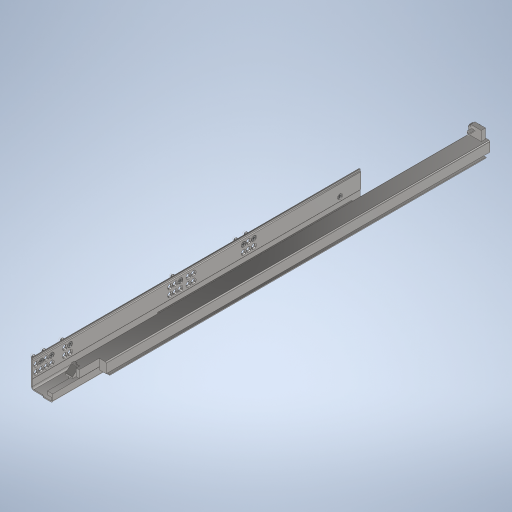
# Autodesk Inventor part: 566H7500B01 Chipboard screws 661.1450.HG 6,3x14,5 top_row L
Saved by Autodesk Inventor 2024 (Build 280153000, 153)
## iProperties
Created: 2019-09-04
Part Number: 566H7500B01 Chipboard screws 661.1450.HG 6,3x14,5 top_row L
Material: Generic
Document SubType Name: Modeling
Designer: RokasM
Density: 1 g/cm^3
Appearance: Default
Author: RokasM
Autodesk Inventor part; units mm, degrees
ref_plane "WP_runner_bottom_displacement_from_facade" through (0, 2, 0) normal (0, 1, 0) x (-1, 0, 0)
sketch "Sketch4" plane through (0, 2, 0) normal (0, 1, 0) x (-1, 0, 0)
  line L0 (0, 47.5) -> (0, 4.8)
  arc A0 (-4.8, 0) -> (0, 4.8) centre (-4.8, 4.8) ccw
  line L1 (-4.8, 0) -> (-36.5, 0)
  arc A1 (-39.3, 2.8) -> (-36.5, 0) centre (-36.5, 2.8) ccw
  line L2 (-39.3, 2.8) -> (-39.3, 13.6)
  line L3 (-39.3, 13.6) -> (-37.5, 13.6)
  line L4 (-37.5, 13.6) -> (-37.5, 2.8)
  arc A2 (-37.5, 2.8) -> (-36.5, 1.8) centre (-36.5, 2.8) ccw
  line L5 (-36.5, 1.8) -> (-4.8, 1.8)
  arc A3 (-4.8, 1.8) -> (-1.8, 4.8) centre (-4.8, 4.8) ccw
  line L6 (-1.8, 4.8) -> (-1.8, 15.95)
  line L7 (-1.8, 15.95) -> (-2.8, 17.25)
  line L8 (-2.8, 17.25) -> (-2.8, 43.75)
  line L9 (-2.8, 43.75) -> (-1.8, 45.05)
  line L10 (-1.8, 45.05) -> (-1.8, 47.5)
  line L11 (-1.8, 47.5) -> (0, 47.5)
  point P0 (0, 0)
  point P1 (-20.65, 0)
  point P2 (0, 26.15)
  dimension "d54" = 2.8
  dimension "d55" = 4.8
  dimension "d56" = 3
  dimension "d57" = 1
  dimension "d58" = 39.3
  dimension "d59" = 47.5
  dimension "d60" = 13.6
  dimension "d61" = 26.5
  dimension "d62" = 2.45
  dimension "d63" = 11.15
  dimension "d64" = 1
  constraints: 24 end point, 8 point on circle, 6 tangent, 5 parallel, 4 centre point, 4 perpendicular, 2 concentric, 2 equal length, 2 midpoint, 1 horizontal, 1 horizontal alignment, 1 vertical alignment
  measures "d54" radius of A1
  measures "d55" radius of A0
  measures "d56" radius of A3
  measures "d57" radius of A2
  measures "d58" distance between parallel lines of L2 L0
  measures "d59" distance between parallel lines of L11 L1
  measures "d60" distance between parallel lines of L3 L1
  measures "d61" distance of L7.end L8.end
  measures "d62" distance of L9.end L10.end
  measures "d63" distance of L6.start L6.end
  measures "d64" distance between parallel lines of L10 L8
extrude "0101_runner_bottom" add sketch "Sketch4" along normal blind 574.8
sketch "Sketch5" plane through (37.5, 2, 2.8) normal (-1, 0, 0) x (0, 0, 1)
  line L0 (10.8, 87) -> (4.9, 87)
  line L1 (4.9, 87) -> (4.9, 0)
  line L2 (4.9, 0) -> (10.8, 0)
  line L3 (10.8, 0) -> (10.8, 87)
  line L4 (10.8, 0) -> (0, 0) projected
  line L5 (10.8, 0) -> (10.8, 574.8) projected
  point P0 (-2.8, -2)
  dimension "d67" = 5.9
  dimension "d68" = 87
  constraints: 8 end point, 2 collinear, 2 parallel, 1 horizontal, 1 perpendicular
  measures "d67" distance of L2.end L1.end
  measures "d68" distance of L1.end L0.end
extrude "0102_runner_bottom_edge" add sketch "Sketch5" along normal blind 7.2
ref_plane "WP_cylinder_start" through (0, 328.35, 0) normal (0, -1, 0) x (1, 0, 0)
sketch "Sketch17" plane through (0, 328.35, 0) normal (0, -1, 0) x (1, 0, 0)
  line L0 (13.3, 1.8) -> (13.3, 6.125)
  arc A0 (21.8, 6.125) -> (13.3, 6.125) centre (17.55, 6.125) ccw
  line L1 (21.8, 6.125) -> (21.8, 3.325)
  line L2 (21.8, 3.325) -> (25, 3.325)
  line L3 (25, 3.325) -> (25, 1.8)
  line L4 (25, 1.8) -> (13.3, 1.8)
  line L5 (4.8, 1.8) -> (36.5, 1.8) projected
  line L6 (0, 4.8) -> (0, 47.5) projected
  point P0 (0, 0)
  dimension "d143" = 4.25
  dimension "d144" = 13.3
  dimension "d145" = 1.525
  dimension "d146" = 3.2
  dimension "d147" = 4.325
  constraints: 10 end point, 4 perpendicular, 2 point on circle, 2 tangent, 1 centre point, 1 collinear
  measures "d143" radius of A0
  measures "d144" distance between parallel lines of L6 L0
  measures "d145" distance between parallel lines of L4 L2
  measures "d146" distance between parallel lines of L1 L3
  measures "d147" distance from line of L4 A0.centre
extrude "0104_cylinder" add sketch "Sketch17" against normal blind 147.5
sketch "Sketch18" plane through (0, 328.35, 0) normal (0, -1, 0) x (1, 0, 0)
  circle A0 centre (17.55, 6.125) radius 0.99
  arc A1 (21.8, 6.125) -> (13.3, 6.125) centre (17.55, 6.125) ccw projected
  point P0 (0, 0)
  point P1 (14.5149, 9.1)
  dimension "d150" = 1.98
  constraints: 1 centre point, 1 concentric
  measures "d150" diameter of A0
extrude "0105_cylinder_piston" add sketch "Sketch18" along normal blind 5.293
sketch "Sketch19" plane through (17.55, 323.057, 6.125) normal (0, -1, 0) x (1, 0, 0)
  line L0 (-3.02, 1.475) -> (4.33, 1.475)
  line L1 (4.33, 1.475) -> (4.33, -4.325)
  line L2 (4.33, -4.325) -> (-3.02, -4.325)
  line L3 (-3.02, -4.325) -> (-3.02, 1.475)
  line L4 (-12.75, -4.325) -> (18.95, -4.325) projected
  line L5 (-17.55, -1.325) -> (-17.55, 41.375) projected
  point P0 (-17.55, -6.125)
  dimension "d153" = 7.35
  dimension "d154" = 5.8
  dimension "d155" = 21.88
  constraints: 8 end point, 2 parallel, 1 collinear, 1 horizontal, 1 perpendicular
  measures "d153" distance between parallel lines of L1 L3
  measures "d154" distance between parallel lines of L2 L0
  measures "d155" distance between parallel lines of L5 L1
extrude "010601_piston_support" add sketch "Sketch19" along normal blind 29.35
sketch "Sketch20" plane through (14.53, 323.057, 7.6) normal (0, 0, 1) x (1, 0, 0)
  line L0 (0.22, -11.475) -> (6.72, -11.475)
  line L1 (6.72, -11.475) -> (6.72, -17.975)
  line L2 (6.72, -17.975) -> (0.22, -17.975)
  line L3 (0.22, -17.975) -> (0.22, -11.475)
  line L4 (7.35, 0) -> (7.35, -29.35) projected
  line L5 (7.35, 0) -> (0, 0) projected
  point P0 (-14.53, -323.057)
  dimension "d158" = 6.5
  dimension "d159" = 6.5
  dimension "d332" = 0.63
  dimension "d333" = 11.475
  constraints: 8 end point, 2 parallel, 1 horizontal, 1 perpendicular
  measures "d158" distance between parallel lines of L2 L0
  measures "d159" distance between parallel lines of L1 L3
  measures "d332" distance between parallel lines of L4 L1
  measures "d333" distance between parallel lines of L5 L0
extrude "010602_piston_support_extrusion" add sketch "Sketch20" along normal blind 4.125
ref_plane "WP_runner_top_displacement_from_runner_bottom" through (0, 48.5, 0) normal (0, -1, 0) x (1, 0, 0)
sketch "Sketch6" plane through (0, 48.5, 0) normal (0, -1, 0) x (1, 0, 0)
  line L0 (33.65, 26.525) -> (38.95, 26.525)
  line L1 (38.95, 26.525) -> (38.95, 13.6)
  line L2 (38.95, 13.6) -> (33.65, 13.6)
  line L3 (33.65, 13.6) -> (33.65, 26.525)
  line L4 (39.3, 13.6) -> (39.3, 2.8) projected
  line L5 (30.3, 13.6) -> (39.3, 13.6) projected
  point P0 (0, 0)
  dimension "d72" = 5.3
  dimension "d73" = 12.925
  dimension "d74" = 0.35
  constraints: 8 end point, 2 parallel, 1 collinear, 1 horizontal, 1 perpendicular
  measures "d72" distance of L1.end L2.end
  measures "d73" distance of L0.end L1.end
  measures "d74" distance between parallel lines of L4 L1
extrude "0201_runner_top" add sketch "Sketch6" against normal blind 35 separate body
sketch "Sketch7" plane through (0, 83.5, 0) normal (0, 1, 0) x (1, 0, 0)
  line L0 (51.05, -26.525) -> (21.35, -26.525)
  line L1 (21.35, -26.525) -> (21.35, -9.125)
  line L2 (21.35, -9.125) -> (51.05, -9.125)
  line L3 (51.05, -9.125) -> (51.05, -26.525)
  line L4 (38.95, -26.525) -> (38.95, -13.6) projected
  line L5 (33.65, -26.525) -> (38.95, -26.525) projected
  point P0 (0, 0)
  dimension "d77" = 29.7
  dimension "d78" = 17.4
  dimension "d79" = 12.1
  constraints: 8 end point, 2 parallel, 1 collinear, 1 horizontal, 1 perpendicular
  measures "d77" distance of L1.end L2.end
  measures "d78" distance of L0.end L1.end
  measures "d79" distance between parallel lines of L4 L3
extrude "0202_runner_top" add sketch "Sketch7" along normal blind 668 bodies 2
sketch "Sketch8" plane through (0, 83.5, 0) normal (0, -1, 0) x (1, 0, 0)
  line L0 (21.35, 9.125) -> (21.35, 26.525)
  line L1 (21.35, 26.525) -> (33.65, 26.525)
  line L2 (33.65, 26.525) -> (33.65, 13.6)
  line L3 (33.65, 13.6) -> (30.3, 13.6)
  line L4 (30.3, 13.6) -> (30.3, 9.125)
  line L5 (30.3, 9.125) -> (21.35, 9.125)
  line L6 (21.35, 26.525) -> (33.65, 26.525) projected
  line L7 (33.65, 26.525) -> (33.65, 13.6) projected
  line L8 (30.3, 13.6) -> (39.3, 13.6) projected
  line L9 (30.3, 7.7) -> (30.3, 13.6) projected
  line L10 (51.05, 9.125) -> (21.35, 9.125) projected
  line L11 (21.35, 9.125) -> (21.35, 26.525) projected
  point P0 (0, 0)
  constraints: 12 end point, 6 collinear
extrude "0203_runner_top" add sketch "Sketch8" along normal blind 26.1 bodies 2
sketch "Sketch9" plane through (0, 57.4, 0) normal (0, -1, 0) x (1, 0, 0)
  line L0 (26.75, 26.525) -> (33.65, 26.525)
  line L1 (33.65, 26.525) -> (33.65, 13.6)
  line L2 (33.65, 13.6) -> (30.3, 13.6)
  line L3 (30.3, 13.6) -> (30.3, 9.125)
  line L4 (30.3, 9.125) -> (26.75, 9.125)
  line L5 (26.75, 9.125) -> (26.75, 26.525)
  line L6 (33.65, 26.525) -> (21.35, 26.525) projected
  line L7 (33.65, 26.525) -> (33.65, 13.6) projected
  line L8 (30.3, 13.6) -> (39.3, 13.6) projected
  line L9 (30.3, 7.7) -> (30.3, 13.6) projected
  line L10 (21.35, 9.125) -> (30.3, 9.125) projected
  point P0 (0, 0)
  dimension "d84" = 6.9
  constraints: 12 end point, 5 collinear, 1 parallel
  measures "d84" distance between parallel lines of L1 L5
extrude "0204_runner_top" add sketch "Sketch9" along normal blind 2.5 bodies 2
sketch "Sketch10" plane through (33.65, 48.5, 26.525) normal (0, 0, 1) x (1, 0, 0)
  line L0 (-10.8, 701.485) -> (11.2, 701.485)
  line L1 (11.2, 701.485) -> (11.2, 694)
  line L2 (11.2, 694) -> (-10.8, 694)
  line L3 (-10.8, 694) -> (-10.8, 701.485)
  line L4 (-12.3, 703) -> (17.4, 703) projected
  line L5 (17.4, 35) -> (17.4, 703) projected
  point P0 (-33.65, -48.5)
  dimension "d87" = 22
  dimension "d88" = 7.485
  dimension "d89" = 1.515
  dimension "d90" = 6.2
  constraints: 8 end point, 2 parallel, 1 horizontal, 1 perpendicular
  measures "d87" distance of L1.end L2.end
  measures "d88" distance of L0.end L1.end
  measures "d89" distance between parallel lines of L4 L0
  measures "d90" distance between parallel lines of L5 L1
extrude "020501_back_pin_support" add sketch "Sketch10" along normal blind 16.7 bodies 2
sketch "Sketch11" plane through (22.85, 742.5, 26.525) normal (0, -1, 0) x (1, 0, 0)
  line L0 (0, 16.7) -> (3.5, 16.7)
  line L1 (3.5, 16.7) -> (3.5, 13.5)
  line L2 (3.5, 13.5) -> (0, 13.5)
  line L3 (0, 13.5) -> (0, 16.7)
  line L4 (0, 16.7) -> (22, 16.7) projected
  line L5 (0, 0) -> (0, 16.7) projected
  point P0 (-22.85, -26.525)
  dimension "d93" = 3.5
  dimension "d94" = 3.2
  constraints: 8 end point, 2 collinear, 2 parallel, 1 horizontal, 1 perpendicular
  measures "d93" distance of L1.end L2.end
  measures "d94" distance of L0.end L1.end
extrude "020502_back_pin_support" cut sketch "Sketch11" against normal up to surface (7.485 mm away) bodies 2
ref_plane "WP_back_pin" through (33.65, 48.5, 38.01) normal (0, 0, 1) x (1, 0, 0)
sketch "Sketch12" plane through (33.65, 48.5, 38.01) normal (0, 0, 1) x (1, 0, 0)
  line L0 (-5.45, 694) -> (0.35, 694)
  line L1 (0.35, 694) -> (0.35, 685.059)
  line L2 (0.35, 685.059) -> (-2.9309, 683.8623)
  arc A0 (-3.611, 684.0377) -> (-2.9309, 683.8623) centre (-3.1433, 684.4447) ccw
  line L3 (-3.611, 684.0377) -> (-5.45, 686.151)
  line L4 (-5.45, 686.151) -> (-5.45, 694)
  line L5 (-7.3, 694) -> (11.2, 694) projected
  line L6 (-7.3, 701.485) -> (-7.3, 694) projected
  point P0 (-33.65, -48.5)
  dimension "d98" = 110.04
  dimension "d99" = 138.97
  dimension "d100" = 0.62
  dimension "d101" = 7.849
  dimension "d102" = 8.941
  dimension "d103" = 5.8
  dimension "d104" = 1.85
  constraints: 10 end point, 2 perpendicular, 2 point on circle, 2 tangent, 1 centre point, 1 collinear
  measures "d98" angle of L1 L2
  measures "d99" angle of L4 L3
  measures "d100" radius of A0
  measures "d101" distance of L3.end L0.start
  measures "d102" distance of L0.end L1.end
  measures "d103" distance between parallel lines of L4 L1
  measures "d104" distance between parallel lines of L6 L4
extrude "020503_back_pin" add sketch "Sketch12" against normal blind 1.485 bodies 2
sketch "Sketch13" plane through (22.85, 749.985, 26.525) normal (0, 1, 0) x (1, 0, 0)
  line L0 (-3.8725, -8) -> (-1.7264, -12.7497)
  line L1 (-1.7264, -12.7497) -> (0.9996, -12.7497)
  line L2 (0.9996, -12.7497) -> (5.8036, -13.7498)
  arc A0 (5.8036, -13.7498) -> (5.8036, -2.2502) centre (11, -8) ccw
  line L3 (5.8036, -2.2502) -> (0.9996, -3.2503)
  line L4 (0.9996, -3.2503) -> (-1.7264, -3.2503)
  line L5 (-1.7264, -3.2503) -> (-3.8725, -8)
  line L6 (22, 0) -> (22, -16.7) projected
  line L7 (22, -16.7) -> (3.5, -16.7) projected
  point P0 (-22.85, 26.525)
  point P1 (-0.3634, -12.7497)
  point P2 (-0.3634, -3.2503)
  dimension "d107" = 7.75
  dimension "d108" = 4.907
  dimension "d109" = 2.726
  dimension "d110" = 5.212
  dimension "d111" = 131.37
  dimension "d112" = 168.24
  dimension "d114" = 168.24
  dimension "d115" = 11
  dimension "d116" = 8.7
  constraints: 12 end point, 3 equal length, 2 midpoint, 2 point on circle, 1 centre point, 1 horizontal, 1 parallel, 1 vertical alignment
  measures "d107" radius of A0
  measures "d108" distance of L1.end L2.end
  measures "d109" distance of L0.end L1.end
  measures "d110" distance of L0.start L0.end
  measures "d111" angle of L5 L0
  measures "d112" angle of L1 L2
  measures "d114" angle of L4 L3
  measures "d115" distance from line of L6 A0.centre
  measures "d116" distance from line of L7 A0.centre
extrude "020601_tilt_adjuster" add sketch "Sketch13" along normal blind 1.48 bodies 2
sketch "Sketch14" plane through (22.85, 749.985, 26.525) normal (0, -1, 0) x (1, 0, 0)
  line L0 (-3.8725, 8) -> (-1.7264, 12.7497)
  line L1 (-1.7264, 12.7497) -> (-0.6564, 12.7497)
  line L2 (-0.6564, 12.7497) -> (-0.6564, 11.9277)
  arc A0 (-0.6564, 11.9277) -> (-0.6564, 4.0723) centre (11, 8) ccw
  line L3 (-0.6564, 4.0723) -> (-0.6564, 3.2503)
  line L4 (-0.6564, 3.2503) -> (-1.7264, 3.2503)
  line L5 (-1.7264, 3.2503) -> (-3.8725, 8)
  line L6 (-1.7264, 12.7497) -> (0, 12.7497) projected
  line L7 (-3.8725, 8) -> (-1.7264, 12.7497) projected
  line L8 (0, 3.2503) -> (-1.7264, 3.2503) projected
  line L9 (-1.7264, 3.2503) -> (-3.8725, 8) projected
  arc A1 (5.8036, 2.2502) -> (5.8036, 13.7498) centre (11, 8) ccw projected
  point P0 (-22.85, -26.525)
  dimension "d119" = 0.822
  dimension "d120" = 1.07
  constraints: 12 end point, 4 collinear, 3 equal length, 2 perpendicular, 2 point on circle, 1 centre point, 1 concentric, 1 parallel
  measures "d119" distance of L1.end L2.end
  measures "d120" distance of L0.end L1.end
extrude "020602_tilt_adjuster" add sketch "Sketch14" along normal blind 4.3 bodies 2
fillet "0207_fillet_runner_top" radius 1.7 2 edges at (21.35, 404.45, 26.525) (51.05, 417.5, 26.525)
ref_plane "WP_runner_middle_displacement_from_runner_bottom" through (0, 89, 0) normal (0, -1, 0) x (1, 0, 0)
sketch "Sketch15" plane through (0, 89, 0) normal (0, -1, 0) x (1, 0, 0)
  line L0 (51.68, 4.205) -> (26.98, 4.205)
  line L1 (26.98, 4.205) -> (26.98, 18.82)
  arc A0 (29.165, 21.005) -> (26.98, 18.82) centre (29.165, 18.82) ccw
  line L2 (29.165, 21.005) -> (43.195, 21.005)
  arc A1 (45.38, 18.82) -> (43.195, 21.005) centre (43.195, 18.82) ccw
  line L3 (45.38, 18.82) -> (45.38, 6.39)
  arc A2 (45.38, 6.39) -> (46.08, 5.69) centre (46.08, 6.39) ccw
  line L4 (46.08, 5.69) -> (51.68, 5.69)
  line L5 (51.68, 5.69) -> (51.68, 4.205)
  line L6 (36.5, 0) -> (4.8, 0) projected
  line L7 (0, 4.8) -> (0, 47.5) projected
  point P0 (0, 0)
  dimension "d125" = 2.185
  dimension "d126" = 2.185
  dimension "d127" = 0.7
  dimension "d128" = 1.485
  dimension "d129" = 24.7
  dimension "d130" = 16.8
  dimension "d131" = 18.4
  dimension "d132" = 4.205
  dimension "d133" = 26.98
  constraints: 12 end point, 6 point on circle, 6 tangent, 3 centre point, 3 perpendicular, 2 parallel, 1 horizontal
  measures "d125" radius of A0
  measures "d126" radius of A1
  measures "d127" radius of A2
  measures "d128" distance between parallel lines of L0 L4
  measures "d129" distance between parallel lines of L1 L5
  measures "d130" distance between parallel lines of L0 L2
  measures "d131" distance between parallel lines of L1 L3
  measures "d132" distance between parallel lines of L6 L0
  measures "d133" distance between parallel lines of L7 L1
extrude "0301_runner_middle" add sketch "Sketch15" against normal blind 655 separate body
sketch "Sketch21" plane through (21.35, 57.4, 9.125) normal (-1, 0, 0) x (0, 0, 1)
  line L0 (-5.8, 0) -> (17.15, 0)
  line L1 (17.15, 0) -> (17.15, -4.54)
  line L2 (17.15, -4.54) -> (15.747, -4.54)
  line L3 (15.747, -4.54) -> (7.1146, -14.9641)
  arc A0 (4.3, -13.95) -> (7.1146, -14.9641) centre (5.89, -13.95) ccw
  line L4 (4.3, -13.95) -> (4.3, -9.3)
  line L5 (4.3, -9.3) -> (-5.8, -9.3)
  line L6 (-5.8, -9.3) -> (-5.8, 0)
  line L7 (0, 0) -> (17.4, 0) projected
  line L8 (17.4, 0) -> (17.4, -2.5) projected
  point P0 (-9.125, -57.4)
  dimension "d164" = 1.59
  dimension "d165" = 22.95
  dimension "d166" = 10.1
  dimension "d167" = 1.403
  dimension "d169" = 4.54
  dimension "d170" = 4.65
  dimension "d171" = 9.3
  dimension "d172" = 8.6324
  dimension "d173" = 0.25
  constraints: 14 end point, 4 perpendicular, 2 point on circle, 2 tangent, 1 centre point, 1 collinear, 1 vertical
  measures "d164" radius of A0
  measures "d165" distance between parallel lines of L6 L1
  measures "d166" distance between parallel lines of L6 L4
  measures "d167" distance of L1.end L2.end
  measures "d169" distance of L0.end L1.end
  measures "d170" distance from line of L5 A0.centre
  measures "d171" distance of L5.end L0.start
  measures "d172" horizontal distance of L2.end L3.end
  measures "d173" distance between parallel lines of L8 L1
extrude "0107_locking_device_lock" add sketch "Sketch21" against normal up to surface (12.3 mm away) bodies 2
sketch "Sketch23" plane through (1.8, 2, 47.5) normal (0, 0, 1) x (1, 0, 0)
  line L0 (-1.8, 2) -> (17.638, 2)
  arc A0 (19.9618, 1) -> (17.638, 2) centre (17.638, -1.2) ccw
  arc A1 (19.9618, 1) -> (22.268, 0) centre (22.2856, 3.2) ccw
  line L1 (22.268, 0) -> (-1.8, 0)
  line L2 (-1.8, 0) -> (-1.8, 2)
  line L3 (3, 0) -> (34.7, 0) projected
  line L4 (-1.8, 0) -> (-1.8, 574.8) projected
  point P0 (-1.8, -2)
  dimension "d185" = 3.2
  dimension "d186" = 3.2
  dimension "d187" = 24.068
  dimension "d188" = 19.438
  dimension "d189" = 2
  constraints: 6 end point, 4 point on circle, 2 centre point, 2 collinear, 2 perpendicular, 2 tangent
  measures "d185" radius of A1
  measures "d186" radius of A0
  measures "d187" distance of L1.start L1.end
  measures "d188" distance of L0.start L0.end
  measures "d189" distance between parallel lines of L0 L1
extrude "0108_runner_bottom_cutout" cut sketch "Sketch23" against normal through all bodies 1
ref_plane "WP_plastic_part_displacement_from_runner_bottom" through (0, 220.65, 0) normal (0, -1, 0) x (1, 0, 0)
sketch "Sketch38" plane through (0, 220.65, 0) normal (0, -1, 0) x (1, 0, 0)
  line L0 (3.2, 9.1) -> (14.53, 9.1)
  line L1 (14.53, 9.1) -> (14.53, 1.8)
  line L2 (14.53, 1.8) -> (3.2, 1.8)
  line L3 (3.2, 1.8) -> (3.2, 9.1)
  line L4 (0, 4.8) -> (0, 47.5) projected
  line L5 (4.8, 1.8) -> (19.438, 1.8) projected
  point P0 (0, 0)
  dimension "d327" = 11.33
  dimension "d328" = 7.3
  dimension "d329" = 14.53
  constraints: 8 end point, 2 parallel, 1 collinear, 1 horizontal, 1 perpendicular
  measures "d327" distance of L1.end L2.end
  measures "d328" distance of L0.end L1.end
  measures "d329" distance between parallel lines of L4 L1
extrude "0103_plastic_part" add sketch "Sketch38" against normal blind 338 bodies 1
ref_plane "WP_mirror" through (0, 289.4, 0) normal (0, -1, 0) x (1, 0, 0)
mirror "0108_mirror_cutout" about plane through (0, 289.4, 0) normal (0, -1, 0) of "0108_runner_bottom_cutout" bodies 1
combine bodies "Combine1" operation type subtract main body 2 bodies to subtract 3 keep tools yes
combine bodies "Combine2" operation type subtract main body 3 bodies to subtract 1 keep tools yes
combine bodies "Combine3" operation type subtract main body 2 bodies to subtract 1 keep tools yes
ref_plane "WP_screw_offset" through (1.305, 4, 4.8) normal (1, 0, 0) x (0, 1, 0)
ref_plane "WP_distance_8h" through (0, 37, 0) normal (0, 1, 0) x (-1, 0, 0)
ref_plane "WP_distance_4h1" through (0, 69, 0) normal (0, 1, 0) x (-1, 0, 0)
ref_plane "WP_distance_6h1" through (0, 261, 0) normal (0, 1, 0) x (-1, 0, 0)
ref_plane "WP_distance_6h2" through (0, 389, 0) normal (0, -1, 0) x (1, 0, 0)
ref_plane "WP_distance_4h2" through (0, 284, 0) normal (0, 1, 0) x (-1, 0, 0)
ref_plane "WP_distance_2h" through (0, 325, 0) normal (0, 1, 0) x (-1, 0, 0)
ref_plane "WP_distance_1h" through (0, 538.8, 0) normal (0, -1, 0) x (1, 0, 0)
sketch "Sketch24" plane through (2.8, 4, 43.75) normal (1, 0, 0) x (0, 0, -1)
  line L0 (43.75, -2) -> (43.75, 572.8) projected
  line L1 (30.15, -2) -> (40.95, -2) projected
  point P0 (43.75, -4)
  point P1 (7.45, 33)
  dimension "d193" = 36.3
  dimension "d194" = 35
  measures "d193" distance from line of L0 point (7.45, 33)
  measures "d194" distance from line of L1 point (7.45, 33)
hole "hole_8_hole_pattern" at (2.8, 37, 36.3) direction (-1, 0, 0) diameter 6.3 end through all countersink diameter 8.99 countersink angle 90 bodies 1
sketch "Sketch26" plane through (2.8, 4, 43.75) normal (1, 0, 0) x (0, 0, -1)
  line L0 (43.75, -2) -> (43.75, 572.8) projected
  line L1 (30.15, -2) -> (40.95, -2) projected
  point P0 (43.75, -4)
  point P1 (7.45, 65)
  dimension "d207" = 36.3
  dimension "d208" = 67
  measures "d207" distance from line of L0 point (7.45, 65)
  measures "d208" distance from line of L1 point (7.45, 65)
hole "hole_4_hole_1st_pattern" at (2.8, 69, 36.3) direction (-1, 0, 0) diameter 6.3 end through all countersink diameter 8.99 countersink angle 90 bodies 1
sketch "Sketch27" plane through (2.8, 4, 43.75) normal (1, 0, 0) x (0, 0, -1)
  line L0 (43.75, -2) -> (43.75, 572.8) projected
  line L1 (30.15, -2) -> (40.95, -2) projected
  point P0 (43.75, -4)
  point P1 (7.45, 257)
  dimension "d216" = 36.3
  dimension "d217" = 259
  measures "d216" distance from line of L0 point (7.45, 257)
  measures "d217" distance from line of L1 point (7.45, 257)
hole "hole_6_hole_1st_pattern" at (2.8, 261, 36.3) direction (-1, 0, 0) diameter 6.3 end through all countersink diameter 8.99 countersink angle 90 bodies 1
sketch "Sketch28" plane through (2.8, 4, 43.75) normal (1, 0, 0) x (0, 0, -1)
  line L0 (43.75, -2) -> (43.75, 572.8) projected
  line L1 (30.15, -2) -> (40.95, -2) projected
  line L2 (53.25, 385) -> (-13.25, 385) projected
  point P0 (43.75, -4)
  point P1 (7.45, 385)
  dimension "d225" = 36.3
  constraints: 1 point on line
  measures "d225" distance from line of L0 point (7.45, 385)
hole "hole_6_hole_2nd_pattern" at (2.8, 389, 36.3) direction (-1, 0, 0) diameter 6.3 end through all countersink diameter 8.99 countersink angle 90 bodies 1
sketch "Sketch29" plane through (2.8, 4, 43.75) normal (1, 0, 0) x (0, 0, -1)
  line L0 (43.75, -2) -> (43.75, 572.8) projected
  line L1 (30.15, -2) -> (40.95, -2) projected
  point P0 (43.75, -4)
  point P1 (7.45, 271)
  dimension "d234" = 36.3
  dimension "d235" = 273
  measures "d234" distance from line of L0 point (7.45, 271)
  measures "d235" distance from line of L1 point (7.45, 271)
hole "hole_4_hole_2nd_pattern" at (2.8, 275, 36.3) direction (-1, 0, 0) diameter 6.3 end through all countersink diameter 8.99 countersink angle 90 bodies 1
sketch "Sketch30" plane through (2.8, 4, 43.75) normal (1, 0, 0) x (0, 0, -1)
  line L0 (43.75, -2) -> (43.75, 572.8) projected
  line L1 (30.15, -2) -> (40.95, -2) projected
  point P0 (43.75, -4)
  point P1 (7.45, 321)
  dimension "d243" = 36.3
  dimension "d244" = 323
  measures "d243" distance from line of L0 point (7.45, 321)
  measures "d244" distance from line of L1 point (7.45, 321)
hole "hole_2_hole_pattern" [suppressed]
sketch "Sketch43" plane through (2.8, 4, 43.75) normal (1, 0, 0) x (0, 0, -1)
  line L0 (53.25, 534.8) -> (-13.25, 534.8) projected
  line L1 (43.75, -2) -> (43.75, 572.8) projected
  point P0 (43.75, -4)
  point P1 (19.45, 534.8)
  dimension "d336" = 24.3
  constraints: 1 point on line
  measures "d336" distance from line of L1 point (19.45, 534.8)
hole "hole_1_hole" at (2.8, 538.8, 24.3) direction (-1, 0, 0) diameter 6.3 end through all countersink diameter 8.99 countersink angle 90 bodies 1
pattern_linear "pattern_8_hole_pattern" count 4 spacing 9 along (0, -1, 0) count 2 spacing 12 along (0, 0, -1) of "hole_8_hole_pattern" bodies 1
pattern_linear "pattern_4_hole_1st_pattern" count 2 spacing 9 along (0, -1, 0) count 2 spacing 12 along (0, 0, -1) of "hole_4_hole_1st_pattern" bodies 1
pattern_linear "pattern_6_hole_1st_pattern" count 3 spacing 9 along (0, -1, 0) count 2 spacing 12 along (0, 0, -1) of "hole_6_hole_1st_pattern" bodies 1
pattern_linear "pattern_6_hole_2nd_pattern" count 3 spacing 9 along (0, -1, 0) count 2 spacing 12 along (0, 0, -1) of "hole_6_hole_2nd_pattern" bodies 1
pattern_linear "pattern_4_hole_2nd_pattern" count 2 spacing 9 along (0, 1, 0) count 2 spacing 12 along (0, 0, -1) of "hole_4_hole_2nd_pattern" bodies 1
pattern_linear "pattern_2_hole_pattern" [suppressed]
sketch "Sketch31" plane through (0, 4, 4.8) normal (-1, 0, 0) x (0, 0, 1)
  circle A0 centre (31.5, 33) radius 2.5
  line L0 (-4.8, 0) -> (-4.8, 570.8) projected
  line L1 (2.9, -2) -> (8.8, -2) projected
  point P0 (-4.8, -4)
  dimension "d285" = 5
  dimension "d286" = 36.3
  dimension "d287" = 35
  constraints: 1 centre point
  measures "d285" diameter of A0
  measures "d286" distance from line of L0 A0.centre
  measures "d287" distance from line of L1 A0.centre
extrude "drill_hole_8_hole_pattern" add sketch "Sketch31" along normal blind 14.5 separate body
sketch "Sketch32" plane through (0, 4, 4.8) normal (-1, 0, 0) x (0, 0, 1)
  circle A0 centre (31.5, 65) radius 2.5
  line L0 (-4.8, 0) -> (-4.8, 570.8) projected
  line L1 (-14.3, -2) -> (52.2, -2) projected
  point P0 (-4.8, -4)
  dimension "d290" = 5
  dimension "d291" = 36.3
  dimension "d292" = 67
  constraints: 1 centre point
  measures "d290" diameter of A0
  measures "d291" distance from line of L0 A0.centre
  measures "d292" distance from line of L1 A0.centre
extrude "drill_hole_4_hole_1st_pattern" add sketch "Sketch32" along normal blind 14.5 separate body
sketch "Sketch33" plane through (0, 4, 4.8) normal (-1, 0, 0) x (0, 0, 1)
  circle A0 centre (31.5, 257) radius 2.5
  line L0 (-4.8, 0) -> (-4.8, 570.8) projected
  line L1 (2.9, -2) -> (8.8, -2) projected
  point P0 (-4.8, -4)
  dimension "d295" = 5
  dimension "d296" = 36.3
  dimension "d297" = 259
  constraints: 1 centre point
  measures "d295" diameter of A0
  measures "d296" distance from line of L0 A0.centre
  measures "d297" distance from line of L1 A0.centre
extrude "drill_hole_6_hole_1st_pattern" add sketch "Sketch33" along normal blind 14.5 separate body
sketch "Sketch34" plane through (0, 4, 4.8) normal (-1, 0, 0) x (0, 0, 1)
  circle A0 centre (31.5, 385) radius 2.5
  line L0 (-4.8, 0) -> (-4.8, 570.8) projected
  line L1 (2.9, -2) -> (8.8, -2) projected
  line L2 (52.2, 385) -> (-14.3, 385) projected
  point P0 (-4.8, -4)
  dimension "d300" = 5
  dimension "d301" = 36.3
  constraints: 1 centre point, 1 point on line
  measures "d300" diameter of A0
  measures "d301" distance from line of L0 A0.centre
extrude "drill_hole_6_hole_2nd_pattern" add sketch "Sketch34" along normal blind 14.5 separate body
sketch "Sketch35" plane through (0, 4, 4.8) normal (-1, 0, 0) x (0, 0, 1)
  circle A0 centre (31.5, 280) radius 2.5
  line L0 (-4.8, 0) -> (-4.8, 570.8) projected
  line L1 (2.9, -2) -> (8.8, -2) projected
  point P0 (-4.8, -4)
  dimension "d305" = 5
  dimension "d306" = 36.3
  dimension "d307" = 282
  constraints: 1 centre point
  measures "d305" diameter of A0
  measures "d306" distance from line of L0 A0.centre
  measures "d307" distance from line of L1 A0.centre
extrude "drill_hole_4_hole_2nd_pattern" [suppressed]
sketch "Sketch36" plane through (0, 4, 4.8) normal (-1, 0, 0) x (0, 0, 1)
  circle A0 centre (31.5, 321) radius 2.5
  line L0 (-4.8, 0) -> (-4.8, 570.8) projected
  line L1 (2.9, -2) -> (8.8, -2) projected
  point P0 (-4.8, -4)
  dimension "d310" = 5
  dimension "d311" = 36.3
  dimension "d312" = 323
  constraints: 1 centre point
  measures "d310" diameter of A0
  measures "d311" distance from line of L0 A0.centre
  measures "d312" distance from line of L1 A0.centre
extrude "drill_hole_2_hole_pattern" [suppressed]
sketch "Sketch45" plane through (1.305, 4, 4.8) normal (1, 0, 0) x (0, 1, 0)
  circle A0 centre (33, 31.5) radius 3
  line L0 (-2, -4.8) -> (572.8, -4.8) projected
  line L1 (33, 52.2) -> (33, -14.3) projected
  point P0 (-4, -4.8)
  dimension "d355" = 6
  dimension "d356" = 36.3
  constraints: 1 centre point, 1 point on line
  measures "d355" diameter of A0
  measures "d356" distance from line of L0 A0.centre
extrude "12_screw_head_8h" add sketch "Sketch45" along normal blind 1 draft 45 separate body
sketch "Sketch47" plane through (1.305, 37, 36.3) normal (-1, 0, 0) x (0, 0, 1)
  circle A0 centre (0, 0) radius 3 projected
  point P0 (-36.3, -37)
extrude "12_screw_thread_8h" add sketch "Sketch47" along normal blind 12.5 bodies 8
sketch "Sketch48" plane through (-11.195, 37, 36.3) normal (-1, 0, 0) x (0, 0, 1)
  circle A0 centre (0, 0) radius 3 projected
  point P0 (-36.3, -37)
extrude "12_screw_tip_8h" add sketch "Sketch48" along normal blind 1 draft -45 bodies 8
sketch "Sketch49" plane through (2.305, 37, 36.3) normal (1, 0, 0) x (0, 0, -1)
  line L0 (-2, -0.5) -> (-2, 0.5)
  line L1 (-2, 0.5) -> (-0.5, 0.5)
  line L2 (-0.5, 0.5) -> (-0.5, 2)
  line L3 (-0.5, 2) -> (0.5, 2)
  line L4 (0.5, 2) -> (0.5, 0.5)
  line L5 (0.5, 0.5) -> (2, 0.5)
  line L6 (2, 0.5) -> (2, -0.5)
  line L7 (2, -0.5) -> (0.5, -0.5)
  line L8 (0.5, -0.5) -> (0.5, -2)
  line L9 (0.5, -2) -> (-0.5, -2)
  line L10 (-0.5, -2) -> (-0.5, -0.5)
  line L11 (-0.5, -0.5) -> (-2, -0.5)
  circle A0 centre (0, 0) radius 4 projected
  point P0 (36.3, -37)
  point P1 (0, 2)
  point P2 (-2, 0)
  dimension "d365" = 1
  dimension "d366" = 1.5
  constraints: 24 end point, 4 collinear, 4 horizontal, 4 perpendicular, 4 vertical, 2 midpoint, 1 horizontal alignment, 1 vertical alignment
  measures "d365" distance of L0.start L0.end
  measures "d366" distance of L0.end L1.end
extrude "12_screw_philips_cut_8h" cut sketch "Sketch49" against normal blind 1 draft -5 contours L0 L1 L2 L3 L4 L5 L6 L7 L8 L9 L10 L11 bodies 8
sketch "Sketch50" plane through (1.305, 4, 4.8) normal (1, 0, 0) x (0, 1, 0)
  circle A0 centre (65, 31.5) radius 3
  line L0 (65, 52.2) -> (65, -14.3) projected
  line L1 (-2, -4.8) -> (572.8, -4.8) projected
  point P0 (-4, -4.8)
  dimension "d369" = 6
  dimension "d370" = 36.3
  constraints: 1 centre point, 1 point on line
  measures "d369" diameter of A0
  measures "d370" distance from line of L1 A0.centre
extrude "13_screw_head_4h1" add sketch "Sketch50" along normal blind 1 draft 45 separate body
sketch "Sketch51" plane through (1.305, 69, 36.3) normal (-1, 0, 0) x (0, 0, 1)
  circle A0 centre (0, 0) radius 3 projected
  point P0 (-36.3, -69)
extrude "13_screw_thread_4h1" add sketch "Sketch51" along normal blind 12.5 bodies 9
sketch "Sketch52" plane through (-11.195, 69, 36.3) normal (-1, 0, 0) x (0, 0, 1)
  circle A0 centre (0, 0) radius 3 projected
  point P0 (-36.3, -69)
extrude "13_screw_tip_4h1" add sketch "Sketch52" along normal blind 1 draft -45 bodies 9
sketch "Sketch53" plane through (2.305, 69, 36.3) normal (1, 0, 0) x (0, 0, -1)
  circle A0 centre (0, 0) radius 4 projected
  line L0 (-2, -0.5) -> (-2, 0.5)
  line L1 (-2, 0.5) -> (-0.5, 0.5)
  line L2 (-0.5, 0.5) -> (-0.5, 2)
  line L3 (-0.5, 2) -> (0.5, 2)
  line L4 (0.5, 2) -> (0.5, 0.5)
  line L5 (0.5, 0.5) -> (2, 0.5)
  line L6 (2, 0.5) -> (2, -0.5)
  line L7 (2, -0.5) -> (0.5, -0.5)
  line L8 (0.5, -0.5) -> (0.5, -2)
  line L9 (0.5, -2) -> (-0.5, -2)
  line L10 (-0.5, -2) -> (-0.5, -0.5)
  line L11 (-0.5, -0.5) -> (-2, -0.5)
  point P0 (36.3, -69)
  point P1 (0, 2)
  point P2 (-2, 0)
  dimension "d377" = 1
  dimension "d378" = 1.5
  constraints: 24 end point, 4 collinear, 4 horizontal, 4 perpendicular, 4 vertical, 2 midpoint, 1 horizontal alignment, 1 vertical alignment
  measures "d377" distance of L0.start L0.end
  measures "d378" distance of L0.end L1.end
extrude "13_screw_philips_cut_4h1" cut sketch "Sketch53" against normal blind 1 draft -5 contours L0 L1 L2 L3 L4 L5 L6 L7 L8 L9 L10 L11 bodies 9
sketch "Sketch54" plane through (1.305, 4, 4.8) normal (1, 0, 0) x (0, 1, 0)
  line L0 (257, 52.2) -> (257, -14.3) projected
  circle A0 centre (257, 31.5) radius 3
  line L1 (-2, -4.8) -> (572.8, -4.8) projected
  point P0 (-4, -4.8)
  dimension "d381" = 6
  dimension "d382" = 36.3
  constraints: 1 centre point, 1 point on line
  measures "d381" diameter of A0
  measures "d382" distance from line of L1 A0.centre
extrude "14_screw_head_6h1" add sketch "Sketch54" along normal blind 1 draft 45 separate body
sketch "Sketch55" plane through (1.305, 261, 36.3) normal (-1, 0, 0) x (0, 0, 1)
  circle A0 centre (0, 0) radius 3 projected
  point P0 (-36.3, -261)
extrude "14_screw_thread_6h1" add sketch "Sketch55" along normal blind 12.5 bodies 10
sketch "Sketch56" plane through (-11.195, 261, 36.3) normal (-1, 0, 0) x (0, 0, 1)
  circle A0 centre (0, 0) radius 3 projected
  point P0 (-36.3, -261)
extrude "14_screw_tip_6h1" add sketch "Sketch56" along normal blind 1 draft -45 bodies 10
sketch "Sketch57" plane through (2.305, 261, 36.3) normal (1, 0, 0) x (0, 0, -1)
  line L0 (-2, -0.5) -> (-2, 0.5)
  line L1 (-2, 0.5) -> (-0.5, 0.5)
  line L2 (-0.5, 0.5) -> (-0.5, 2)
  line L3 (-0.5, 2) -> (0.5, 2)
  line L4 (0.5, 2) -> (0.5, 0.5)
  line L5 (0.5, 0.5) -> (2, 0.5)
  line L6 (2, 0.5) -> (2, -0.5)
  line L7 (2, -0.5) -> (0.5, -0.5)
  line L8 (0.5, -0.5) -> (0.5, -2)
  line L9 (0.5, -2) -> (-0.5, -2)
  line L10 (-0.5, -2) -> (-0.5, -0.5)
  line L11 (-0.5, -0.5) -> (-2, -0.5)
  circle A0 centre (0, 0) radius 4 projected
  point P0 (36.3, -261)
  point P1 (-2, 0)
  point P2 (0, 2)
  dimension "d389" = 1
  dimension "d390" = 1.5
  constraints: 24 end point, 4 collinear, 4 horizontal, 4 perpendicular, 4 vertical, 2 midpoint, 1 horizontal alignment, 1 vertical alignment
  measures "d389" distance of L0.start L0.end
  measures "d390" distance of L0.end L1.end
extrude "14_screw_philips_cut_6h1" cut sketch "Sketch57" against normal blind 1 draft -5 contours L0 L1 L2 L3 L4 L5 L6 L7 L8 L9 L10 L11 bodies 10
sketch "Sketch58" plane through (1.305, 4, 4.8) normal (1, 0, 0) x (0, 1, 0)
  circle A0 centre (385, 31.5) radius 3
  line L0 (385, -14.3) -> (385, 52.2) projected
  line L1 (-2, -4.8) -> (572.8, -4.8) projected
  point P0 (-4, -4.8)
  dimension "d393" = 6
  dimension "d394" = 36.3
  constraints: 1 centre point, 1 point on line
  measures "d393" diameter of A0
  measures "d394" distance from line of L1 A0.centre
extrude "15_screw_head_6h2" add sketch "Sketch58" along normal blind 1 draft 45 separate body
sketch "Sketch59" plane through (1.305, 389, 36.3) normal (-1, 0, 0) x (0, 0, 1)
  circle A0 centre (0, 0) radius 3 projected
  point P0 (-36.3, -389)
extrude "15_screw_thread_6h2" add sketch "Sketch59" along normal blind 12.5 bodies 11
sketch "Sketch60" plane through (-11.195, 389, 36.3) normal (-1, 0, 0) x (0, 0, 1)
  circle A0 centre (0, 0) radius 3 projected
  point P0 (-36.3, -389)
extrude "15_screw_tip_6h2" add sketch "Sketch60" along normal blind 1 draft -45 bodies 11
sketch "Sketch61" plane through (2.305, 389, 36.3) normal (1, 0, 0) x (0, 0, -1)
  line L0 (-2, -0.5) -> (-2, 0.5)
  line L1 (-2, 0.5) -> (-0.5, 0.5)
  line L2 (-0.5, 0.5) -> (-0.5, 2)
  line L3 (-0.5, 2) -> (0.5, 2)
  line L4 (0.5, 2) -> (0.5, 0.5)
  line L5 (0.5, 0.5) -> (2, 0.5)
  line L6 (2, 0.5) -> (2, -0.5)
  line L7 (2, -0.5) -> (0.5, -0.5)
  line L8 (0.5, -0.5) -> (0.5, -2)
  line L9 (0.5, -2) -> (-0.5, -2)
  line L10 (-0.5, -2) -> (-0.5, -0.5)
  line L11 (-0.5, -0.5) -> (-2, -0.5)
  circle A0 centre (0, 0) radius 4 projected
  point P0 (36.3, -389)
  point P1 (0, 2)
  point P2 (-2, 0)
  dimension "d401" = 1
  dimension "d402" = 1.5
  constraints: 24 end point, 4 collinear, 4 horizontal, 4 perpendicular, 4 vertical, 2 midpoint, 1 horizontal alignment, 1 vertical alignment
  measures "d401" distance of L0.start L0.end
  measures "d402" distance of L0.end L1.end
extrude "15_screw_philips_cut_6h2" cut sketch "Sketch61" against normal blind 1 draft -5 contours L0 L1 L2 L3 L4 L5 L6 L7 L8 L9 L10 L11 bodies 11
sketch "Sketch62" plane through (1.305, 4, 4.8) normal (1, 0, 0) x (0, 1, 0)
  line L0 (280, 52.2) -> (280, -14.3) projected
  circle A0 centre (280, 31.5) radius 3
  line L1 (-2, -4.8) -> (572.8, -4.8) projected
  point P0 (-4, -4.8)
  dimension "d406" = 6
  dimension "d407" = 36.3
  constraints: 1 centre point, 1 point on line
  measures "d406" diameter of A0
  measures "d407" distance from line of L1 A0.centre
extrude "16_screw_head_4h2" [suppressed]
sketch "Sketch63" plane through (0.055, 284, 24.3) normal (-1, 0, 0) x (0, 0, 1)
  circle A0 centre (0, 0) radius 1.75 projected
  point P0 (-24.3, -284)
extrude "16_screw_thread_4h2" [suppressed]
sketch "Sketch64" plane through (-9.195, 284, 24.3) normal (-1, 0, 0) x (0, 0, 1)
  circle A0 centre (0, 0) radius 1.75 projected
  point P0 (-24.3, -284)
extrude "16_screw_tip_4h2" [suppressed]
sketch "Sketch65" plane through (1.805, 284, 24.3) normal (1, 0, 0) x (0, 0, -1)
  line L0 (-2, -0.5) -> (-2, 0.5)
  line L1 (-2, 0.5) -> (-0.5, 0.5)
  line L2 (-0.5, 0.5) -> (-0.5, 2)
  line L3 (-0.5, 2) -> (0.5, 2)
  line L4 (0.5, 2) -> (0.5, 0.5)
  line L5 (0.5, 0.5) -> (2, 0.5)
  line L6 (2, 0.5) -> (2, -0.5)
  line L7 (2, -0.5) -> (0.5, -0.5)
  line L8 (0.5, -0.5) -> (0.5, -2)
  line L9 (0.5, -2) -> (-0.5, -2)
  line L10 (-0.5, -2) -> (-0.5, -0.5)
  line L11 (-0.5, -0.5) -> (-2, -0.5)
  circle A0 centre (0, 0) radius 3.5 projected
  point P0 (24.3, -284)
  point P1 (0, 2)
  point P2 (-2, 0)
  dimension "d414" = 1
  dimension "d415" = 1.5
  constraints: 24 end point, 4 collinear, 4 horizontal, 4 perpendicular, 4 vertical, 2 midpoint, 1 horizontal alignment, 1 vertical alignment
  measures "d414" distance of L0.start L0.end
  measures "d415" distance of L0.end L1.end
extrude "16_screw_philips_cut_4h2" [suppressed]
sketch "Sketch66" plane through (1.305, 4, 4.8) normal (1, 0, 0) x (0, 1, 0)
  line L0 (321, 52.2) -> (321, -14.3) projected
  circle A0 centre (321, 31.5) radius 3
  line L1 (-2, -4.8) -> (572.8, -4.8) projected
  point P0 (-4, -4.8)
  dimension "d419" = 6
  dimension "d420" = 36.3
  constraints: 1 centre point, 1 point on line
  measures "d419" diameter of A0
  measures "d420" distance from line of L1 A0.centre
extrude "17_screw_head_2h" [suppressed]
sketch "Sketch67" plane through (0.055, 325, 36.3) normal (-1, 0, 0) x (0, 0, 1)
  circle A0 centre (0, 0) radius 1.75 projected
  point P0 (-36.3, -325)
extrude "17_screw_thread_2h" [suppressed]
sketch "Sketch68" plane through (-9.195, 325, 36.3) normal (-1, 0, 0) x (0, 0, 1)
  circle A0 centre (0, 0) radius 1.75 projected
  point P0 (-36.3, -325)
extrude "17_screw_tip_2h" [suppressed]
sketch "Sketch69" plane through (1.805, 325, 36.3) normal (1, 0, 0) x (0, 0, -1)
  line L0 (-2, -0.5) -> (-2, 0.5)
  line L1 (-2, 0.5) -> (-0.5, 0.5)
  line L2 (-0.5, 0.5) -> (-0.5, 2)
  line L3 (-0.5, 2) -> (0.5, 2)
  line L4 (0.5, 2) -> (0.5, 0.5)
  line L5 (0.5, 0.5) -> (2, 0.5)
  line L6 (2, 0.5) -> (2, -0.5)
  line L7 (2, -0.5) -> (0.5, -0.5)
  line L8 (0.5, -0.5) -> (0.5, -2)
  line L9 (0.5, -2) -> (-0.5, -2)
  line L10 (-0.5, -2) -> (-0.5, -0.5)
  line L11 (-0.5, -0.5) -> (-2, -0.5)
  circle A0 centre (0, 0) radius 3.5 projected
  point P0 (36.3, -325)
  point P1 (-2, 0)
  point P2 (0, 2)
  dimension "d427" = 1
  dimension "d428" = 1.5
  constraints: 24 end point, 4 collinear, 4 horizontal, 4 perpendicular, 4 vertical, 2 midpoint, 1 horizontal alignment, 1 vertical alignment
  measures "d427" distance of L0.start L0.end
  measures "d428" distance of L0.end L1.end
extrude "17_screw_philips_cut__2h" [suppressed]
pattern_linear "second_drill_hole_8_hole_pattern" count 2 spacing 18 along (0, -1, 0) bodies 4 8
pattern_linear "second_drill_hole_6_hole_1st_pattern" [suppressed]
pattern_linear "second_drill_hole_6_hole_2nd_pattern" count 2 spacing 18 along (0, -1, 0) bodies 7 11
sketch "Sketch44" plane through (0, 4, 4.8) normal (-1, 0, 0) x (0, 0, 1)
  line L0 (52.2, 534.8) -> (-14.3, 534.8) projected
  circle A0 centre (19.5, 534.8) radius 0.5
  line L1 (-4.8, 0) -> (-4.8, 570.8) projected
  point P0 (-4.8, -4)
  dimension "d344" = 1
  dimension "d345" = 24.3
  constraints: 1 centre point, 1 point on line
  measures "d344" diameter of A0
  measures "d345" distance from line of L1 A0.centre
extrude "drill_hole_1_hole" add sketch "Sketch44" along normal blind 10 separate body
sketch "Sketch37" plane through (44.85, 742.5, 26.525) normal (0, -1, 0) x (1, 0, 0)
  line L0 (-16.65, 11.485) -> (-10.85, 11.485) construction
  line L1 (-10.85, 10) -> (-16.65, 10) construction
  circle A0 centre (-13.75, 10.7425) radius 3
  line L2 (-10.85, 11.485) -> (-10.85, 10) projected
  point P0 (-44.85, -26.525)
  point P1 (-10.85, 10.7425)
  point P2 (-13.75, 11.485)
  dimension "d321" = 6
  constraints: 2 midpoint, 1 centre point, 1 horizontal alignment, 1 vertical alignment
  measures "d321" diameter of A0
extrude "drill_hole_back_pin" add sketch "Sketch37" along normal blind 10 separate body
ref_plane "WP_screw_1h" through (0.055, 4, 4.8) normal (-1, 0, 0) x (0, 0, 1)
sketch "Sketch70" plane through (0.055, 4, 4.8) normal (1, 0, 0) x (0, 1, 0)
  line L0 (534.8, -14.3) -> (534.8, 52.2) projected
  circle A0 centre (534.8, 19.5) radius 1.75
  line L1 (-2, -4.8) -> (572.8, -4.8) projected
  point P0 (-4, -4.8)
  dimension "d431" = 3.5
  dimension "d432" = 24.3
  constraints: 1 centre point, 1 point on line
  measures "d431" diameter of A0
  measures "d432" distance from line of L1 A0.centre
extrude "18_screw_head_1h" add sketch "Sketch70" along normal blind 1.75 draft 45 separate body
sketch "Sketch71" plane through (0.055, 538.8, 24.3) normal (-1, 0, 0) x (0, 0, 1)
  circle A0 centre (0, 0) radius 1.75 projected
  point P0 (-24.3, -538.8)
extrude "18_screw_thread_1h" add sketch "Sketch71" along normal blind 9.25 bodies 1
sketch "Sketch72" plane through (-9.195, 538.8, 24.3) normal (-1, 0, 0) x (0, 0, 1)
  circle A0 centre (0, 0) radius 1.75 projected
  point P0 (-24.3, -538.8)
extrude "18_screw_tip_1h" add sketch "Sketch72" along normal blind 5 draft -18 bodies 1
sketch "Sketch73" plane through (1.805, 538.8, 24.3) normal (1, 0, 0) x (0, 0, -1)
  line L0 (-2, -0.5) -> (-2, 0.5)
  line L1 (-2, 0.5) -> (-0.5, 0.5)
  line L2 (-0.5, 0.5) -> (-0.5, 2)
  line L3 (-0.5, 2) -> (0.5, 2)
  line L4 (0.5, 2) -> (0.5, 0.5)
  line L5 (0.5, 0.5) -> (2, 0.5)
  line L6 (2, 0.5) -> (2, -0.5)
  line L7 (2, -0.5) -> (0.5, -0.5)
  line L8 (0.5, -0.5) -> (0.5, -2)
  line L9 (0.5, -2) -> (-0.5, -2)
  line L10 (-0.5, -2) -> (-0.5, -0.5)
  line L11 (-0.5, -0.5) -> (-2, -0.5)
  circle A0 centre (0, 0) radius 3.5 projected
  point P0 (24.3, -538.8)
  point P1 (0, 2)
  point P2 (-2, 0)
  dimension "d440" = 1
  dimension "d441" = 1.5
  constraints: 24 end point, 4 collinear, 4 horizontal, 4 perpendicular, 4 vertical, 2 midpoint, 1 horizontal alignment, 1 vertical alignment
  measures "d440" distance of L0.start L0.end
  measures "d441" distance of L0.end L1.end
extrude "18_screw_philips_cut_1h" cut sketch "Sketch73" against normal blind 1 draft -5 contours L0 L1 L2 L3 L4 L5 L6 L7 L8 L9 L10 L11 bodies 14
mirror "mirror_runner_8h_4h1_pin" [suppressed]
mirror "mirror_6h1" [suppressed]
mirror "mirror_6h2" [suppressed]
mirror "mirror_4h2" [suppressed]
mirror "mirror_2h" [suppressed]
ref_plane "Work Plane8" through (0, 289.4, 0) normal (0, -1, 0) x (1, 0, 0)
equation "\"d58\" = runner_bottom_width"
equation "\"d59\" = runner_bottom_height"
equation "\"d60\" = runner_bottom_inside_edge"
equation "\"d65\" = runner_bottom_length"
equation "\"d148\" = cylinder_end - cylinder_start"
equation "\"d80\" = runner_top_length"
equation "\"d114\" = d112"
equation "\"d126\" = d125"
equation "\"d134\" = runner_middle_length"
equation "\"runner_bottom_width\" = 39.3"
equation "\"runner_bottom_height\" = 47.5"
equation "\"displacement_between_facade_and_runner\" = 2"
equation "\"distance_runner_bottom_to_8_hole_pattern\" = 35"
equation "\"distance_runner_bottom_to_4_hole_1st_pattern\" = 67"
equation "\"distance_runner_bottom_to_6_hole_1st_pattern\" = 259"
equation "\"distance_runner_bottom_to_6_hole_2nd_pattern\" = 387"
equation "\"distance_runner_bottom_to_4_hole_2nd_pattern\" = 273"
equation "\"distance_runner_bottom_to_2_hole_pattern\" = 323"
equation "\"hole_horizontal_displacement\" = 9"
equation "\"hole_vertical_dsplacement\" = 12"
equation "\"bottom_row\" = 24.3"
equation "\"hole_diameter\" = 6.3"
equation "\"bolt_head_diameter\" = 8.99"
equation "\"pin_hole_diameter\" = 6"
equation "\"NL560_30_32\" = 280.8"
equation "\"NL560_38\" = 355.9"
equation "\"NL560_40_42_45_48_50_52_55\" = 383.9"
equation "\"NL560_60\" = 428"
equation "\"NL566_45_50_52_55_58\" = 421"
equation "\"NL566_60\" = 445.1"
equation "\"NL566_65\" = 470.1"
equation "\"NL566_70\" = 495.1"
equation "\"NL566_75\" = 574.8"
equation "\"runner_bottom_length\" = 574.8"
equation "\"runner_bottom_inside_edge\" = 13.6"
equation "\"d23\" = displacement_between_facade_and_runner"
equation "\"runner_bottom_start\" = 87"
equation "\"LD_plane\" = 46.5"
equation "\"d71\" = -LD_plane"
equation "\"runner_top_length\" = 668"
equation "\"d124\" = -runner_bottom_start"
equation "\"runner_middle_length\" = 655"
equation "\"plastic_part_start\" = 218.65"
equation "\"plastic_part_end\" = 556.65"
equation "\"cylinder_start\" = 326.35"
equation "\"cylinder_end\" = 473.85"
equation "\"d142\" = -cylinder_start"
equation "\"drill_diameter\" = 5"
equation "\"drill_depth\" = 14.5"
equation "\"top_row\" = 36.3"
equation "\"drilling_row\" = 36.3"
equation "\"distance_runner_bottom_to_1_hole\" = 536.8"
equation "\"screw_plane_offset\" = 1.305"
equation "\"screw_thread_diameter\" = 6"
equation "\"screw_thread_length\" = 12.5"
equation "\"screw_head_length\" = 1"
equation "\"screw_tip_length\" = 1"
equation "\"screw_tip_angle\" = 45deg"
